plate_holder (Autodesk Fusion 360 design; units mm, degrees)
Autodesk Fusion 360 part; units mm, degrees
sketch "Sketch1" plane through (0, 0, 0) normal (0, 1, 0) x (1, 0, 0)
  line L0 (-177.8, -120.65) -> (0, -120.65)
  line L1 (0, -120.65) -> (0, 0)
  line L2 (0, 0) -> (-177.8, 0)
  line L3 (-177.8, 0) -> (-177.8, -120.65)
  circle A0 centre (-177.8, -120.65) radius 3.175
  circle A1 centre (-177.8, 0) radius 3.175
  circle A2 centre (0, 0) radius 3.175
  circle A3 centre (0, -120.65) radius 3.175
  line L4 (-158.9, -97.1) -> (-18.9, -97.1)
  line L5 (-18.9, -97.1) -> (-18.9, -72.1)
  line L6 (-18.9, -72.1) -> (-158.9, -72.1)
  line L7 (-158.9, -72.1) -> (-158.9, -97.1)
  line L8 (-158.9, -48.55) -> (-18.9, -48.55)
  line L9 (-18.9, -48.55) -> (-18.9, -23.55)
  line L10 (-18.9, -23.55) -> (-158.9, -23.55)
  line L11 (-158.9, -23.55) -> (-158.9, -48.55)
  line L12 (-180.975, -120.65) -> (-174.625, -120.65)
  line L13 (-174.625, -120.65) -> (-174.625, 0)
  line L14 (-174.625, 0) -> (-180.975, 0)
  line L15 (-180.975, 0) -> (-180.975, -120.65)
  line L16 (3.175, -120.65) -> (-3.175, -120.65)
  line L17 (-3.175, -120.65) -> (-3.175, 0)
  line L18 (-3.175, 0) -> (3.175, 0)
  line L19 (3.175, 0) -> (3.175, -120.65)
  line L20 (0, 0) -> (0, 3.175)
  line L21 (0, 3.175) -> (-177.8, 3.175)
  line L22 (-177.8, 3.175) -> (-177.8, -3.175)
  line L23 (-177.8, -3.175) -> (0, -3.175)
  line L24 (0, -3.175) -> (0, 3.175)
  line L25 (0, -120.65) -> (0, -123.825)
  line L26 (0, -123.825) -> (-177.8, -123.825)
  line L27 (-177.8, -123.825) -> (-177.8, -117.475)
  line L28 (-177.8, -117.475) -> (0, -117.475)
  line L29 (0, -117.475) -> (0, -123.825)
  line L30 (-177.8, -117.475) -> (-174.625, -117.475)
  line L31 (-174.625, -117.475) -> (-174.625, -120.65)
  line L32 (-174.625, -120.65) -> (-177.8, -120.65)
  line L33 (-177.8, -120.65) -> (-177.8, -117.475)
  line L34 (-158.9, -89.1) -> (-18.9, -89.1)
  line L35 (-18.9, -89.1) -> (-18.9, -80.1)
  line L36 (-18.9, -80.1) -> (-158.9, -80.1)
  line L37 (-158.9, -80.1) -> (-158.9, -89.1)
  line L38 (-150.9, -97.1) -> (-26.9, -97.1)
  line L39 (-26.9, -97.1) -> (-26.9, -72.1)
  line L40 (-26.9, -72.1) -> (-150.9, -72.1)
  line L41 (-150.9, -72.1) -> (-150.9, -97.1)
  line L42 (-177.8, -117.475) -> (-158.9, -89.1)
  line L43 (-174.625, -120.65) -> (-150.9, -97.1)
  line L44 (-26.9, -97.1) -> (-3.175, -120.65)
  line L45 (-18.9, -89.1) -> (0, -117.475)
  line L46 (-158.9, -40.55) -> (-18.9, -40.55)
  line L47 (-18.9, -40.55) -> (-18.9, -31.55)
  line L48 (-18.9, -31.55) -> (-158.9, -31.55)
  line L49 (-158.9, -31.55) -> (-158.9, -40.55)
  line L50 (-150.9, -48.55) -> (-26.9, -48.55)
  line L51 (-26.9, -48.55) -> (-26.9, -23.55)
  line L52 (-26.9, -23.55) -> (-150.9, -23.55)
  line L53 (-150.9, -23.55) -> (-150.9, -48.55)
  line L54 (-18.9, -31.55) -> (0, -3.175)
  line L55 (-26.9, -23.55) -> (-3.175, 0)
  line L56 (-158.9, -31.55) -> (-177.8, -3.175)
  line L57 (-150.9, -23.55) -> (-174.625, 0)
  line L58 (0, -60.325) -> (-177.8, -60.325)
  line L59 (-158.9, -40.55) -> (-174.625, -51.5608)
  line L60 (-150.9, -48.55) -> (-167.7164, -60.325)
  line L61 (-150.9, -72.1) -> (-167.7164, -60.325)
  line L62 (-158.9, -80.1) -> (-174.625, -69.0892)
  line L63 (-18.9, -80.1) -> (-3.175, -69.0892)
  line L64 (-18.9, -40.55) -> (-3.175, -51.5608)
  line L65 (-26.9, -48.55) -> (-10.0836, -60.325)
  line L66 (-26.9, -72.1) -> (-10.0836, -60.325)
  line L67 (-150.9, -97.1) -> (-130.6753, -117.475)
  line L68 (-136.8099, -97.1) -> (-116.5852, -117.475)
  line L69 (-116.5852, -117.475) -> (-101.3782, -97.1)
  line L70 (-26.9, -97.1) -> (-47.1247, -117.475)
  line L71 (-40.9901, -97.1) -> (-61.2148, -117.475)
  line L72 (-61.2148, -117.475) -> (-76.4218, -97.1)
  line L73 (-104.107, -117.475) -> (-88.9, -97.1)
  line L74 (-88.9, -97.1) -> (-73.693, -117.475)
  line L75 (-140.9, -72.1) -> (-18.4918, -54.4375)
  line L76 (-159.3082, -66.2125) -> (-36.9, -48.55)
  line L77 (-18.4918, -66.2125) -> (-140.9, -48.55)
  line L78 (-159.3082, -54.4375) -> (-36.9, -72.1)
  line L79 (-150.9, -23.55) -> (-130.6753, -3.175)
  line L80 (-136.8099, -23.55) -> (-116.5852, -3.175)
  line L81 (-116.5852, -3.175) -> (-101.3782, -23.55)
  line L82 (-104.107, -3.175) -> (-88.9, -23.55)
  line L83 (-88.9, -23.55) -> (-73.693, -3.175)
  line L84 (-61.2148, -3.175) -> (-76.4218, -23.55)
  line L85 (-40.9901, -23.55) -> (-61.2148, -3.175)
  line L86 (-26.9, -23.55) -> (-47.1247, -3.175)
  dimension "d1" = 177.8
  dimension "d2" = 120.65
  dimension "d3" = 6.35
  dimension "d4" = 6.35
  dimension "d6" = 6.35
  dimension "d7" = 6.35
  dimension "d10" = 25
  dimension "d11" = 25
  dimension "d12" = 140
  dimension "d13" = 140
  dimension "d14" = 23.55
  dimension "d15" = 23.55
  dimension "d16" = 18.9
  dimension "d17" = 18.9
  dimension "d18" = 8
  dimension "d19" = 8
  dimension "d20" = 8
  dimension "d21" = 8
  dimension "d22" = 8
  dimension "d23" = 8
  dimension "d24" = 8
  dimension "d25" = 8
  dimension "d26" = 125
  dimension "d27" = 125
  dimension "d28" = 10
  dimension "d30" = 45.212
  dimension "d31" = 45.212
  dimension "d32" = 10
  dimension "d33" = 10
  dimension "d34" = 10
  dimension "d35" = 10
  dimension "d36" = 10
  dimension "d37" = 10
  dimension "d38" = 10
  constraint horizontal L0
  constraint vertical L1
  constraint horizontal L2
  constraint vertical L3
  constraint coincident L1.end L2.start
  constraint coincident L0.start L3.end
  constraint coincident L2.end L3.start
  constraint coincident L0.end L1.start
  constraint horizontal L4
  constraint vertical L5
  constraint horizontal L6
  constraint vertical L7
  constraint horizontal L8
  constraint vertical L9
  constraint horizontal L10
  constraint vertical L11
  constraint horizontal L12
  constraint vertical L13
  constraint horizontal L14
  constraint vertical L15
  constraint coincident L2 L13.end
  constraint coincident A1 L13.end
  constraint coincident A0 L12.start
  constraint horizontal L16
  constraint vertical L17
  constraint horizontal L18
  constraint vertical L19
  constraint coincident A2 L17.end
  constraint coincident L2 L17.end
  constraint coincident A3 L16.start
  constraint perpendicular L2 L20
  constraint horizontal L21
  constraint vertical L22
  constraint horizontal L23
  constraint vertical L24
  constraint coincident A1 L22.end
  constraint coincident L3 L22.end
  constraint coincident A2 L20.end
  constraint coincident L20 L21.start
  constraint coincident A3 L25.end
  constraint perpendicular L0 L25
  constraint horizontal L26
  constraint vertical L27
  constraint horizontal L28
  constraint vertical L29
  constraint coincident A0 L27.end
  constraint coincident L3 L27.end
  constraint horizontal L30
  constraint vertical L31
  constraint horizontal L32
  constraint vertical L33
  constraint horizontal L34
  constraint vertical L35
  constraint horizontal L36
  constraint vertical L37
  constraint coincident L5 L35.end
  constraint coincident L7 L34.start
  constraint horizontal L38
  constraint vertical L39
  constraint horizontal L40
  constraint vertical L41
  constraint coincident L6 L39.end
  constraint coincident L4 L38.start
  constraint horizontal L46
  constraint vertical L47
  constraint horizontal L48
  constraint vertical L49
  constraint coincident L9 L47.end
  constraint coincident L11 L46.start
  constraint horizontal L50
  constraint vertical L51
  constraint horizontal L52
  constraint vertical L53
  constraint coincident L10 L51.end
  constraint coincident L8 L50.start
  constraint midpoint L1 L58.start
  constraint midpoint L3 L58.end
  constraint coincident L0.start L12
  constraint coincident L0.end L16
  constraint coincident L13 L59.end
  constraint coincident L58 L60.end
  constraint coincident L13 L62.end
  constraint parallel L61 L62
  constraint coincident L17 L63.end
  constraint parallel L60 L63
  constraint coincident L17 L64.end
  constraint parallel L62 L64
  constraint coincident L58 L65.end
  constraint parallel L64 L65
  constraint coincident L28 L67.end
  constraint perpendicular L43 L67
  constraint coincident L38 L68.start
  constraint coincident L28 L68.end
  constraint parallel L67 L68
  constraint coincident L4 L69.end
  constraint coincident L28 L70.end
  constraint coincident L38 L71.start
  constraint coincident L28 L71.end
  constraint coincident L4 L72.end
  constraint coincident L28 L73.start
  constraint midpoint L38 L73.end
  constraint coincident L28 L74.end
  constraint parallel L72 L74
  constraint parallel L70 L71
  constraint parallel L69 L73
  constraint coincident L40 L75.start
  constraint midpoint L65 L75.end
  constraint midpoint L61 L76.start
  constraint coincident L8 L76.end
  constraint midpoint L66 L77.start
  constraint coincident L50 L77.end
  constraint midpoint L60 L78.start
  constraint coincident L6 L78.end
  constraint symmetric L38.start L58 L52.end
  constraint symmetric L38.end L58 L51.end
  constraint symmetric L58 L67.end L79.end
  constraint symmetric L58 L68.start L80.start
  constraint symmetric L58 L68.end L80.end
  constraint symmetric L58 L69.end L81.end
  constraint symmetric L58 L70.end L86.end
  constraint symmetric L58 L71.start L85.start
  constraint symmetric L58 L71.end L84.start
  constraint symmetric L58 L72.end L84.end
  constraint symmetric L58 L73.start L82.start
  constraint symmetric L58 L73.end L82.end
  constraint symmetric L58 L74.end L83.end
  measures "d1" distance of L0.start L0.end
  measures "d2" distance of L0.start L2.end
  measures "d3" diameter of A0
  measures "d4" diameter of A3
  measures "d6" diameter of A2
  measures "d7" diameter of A1
  measures "d10" distance of L4.start L6.end
  measures "d11" distance of L8.start L10.end
  measures "d12" distance of L4.start L4.end
  measures "d13" distance of L8.start L8.end
  measures "d14" distance of L0 L4
  measures "d15" distance of L6 L8
  measures "d16" distance of L3 L7
  measures "d17" distance of L3 L11
  measures "d18" distance of L37 L41
  measures "d19" distance of L35 L39
  measures "d20" distance of L9 L51
  measures "d21" distance of L11 L53
  measures "d22" distance of L34 L38
  measures "d23" distance of L36 L40
  measures "d24" distance of L46 L50
  measures "d25" distance of L48 L52
  measures "d26" angle of L13 L62
  measures "d27" angle of L13 L59
  measures "d28" distance of L67 L68
  measures "d30" angle of L38 L70
  measures "d31" angle of L4 L67
  measures "d32" distance of L69 L73
  measures "d33" distance of L70 L71
  measures "d34" distance of L72 L74
  measures "d35" distance of L40.end L75.start
  measures "d36" distance of L50.end L76.end
  measures "d37" distance of L39.end L78.end
  measures "d38" distance of L50.start L77.end
extrude "Extrude1" add sketch "Sketch1" along normal blind 5 contours L0 L3 A0 L12 L27 L32 L33 | L3 A0 L12 L27 L33 | A0 L12 L27 | L0 A0 L12 L27 L32 | L0 L1 A3 L16 L29 | L0 A3 L16 L25 L29 | L3 A1 L14 L22 | A1 L14 L22 | A3 L16 L25 L29 | L1 A3 L16 L29 | L2 L3 A1 L14 L22 | L2 A1 L14 L22 | L2 A2 L18 L20 L24 | A2 L18 L20 L24 | L1 A2 L18 L24 | L1 L2 A2 L18 L24 makes body 1 at (3.1592, 1.6667, 0.3161) makes body 2 at (-176.3515, 3.3333, 2.8253) makes body 3 at (3.1592, 3.3333, 120.3339) makes body 4 at (-179.6534, 3.3333, 118.0721)
extrude "Extrude2" add sketch "Sketch1" 1 faces at (0.6951, 0, 119.3529) against normal blind 4 contours L0 L3 A0 L12 L27 L32 L33 | L3 A0 L12 L27 L33 | A0 L12 L27 | L0 A0 L12 L27 L32 | L0 L28 L43 L44 | L0 A0 A3 L26 | A0 L13 L28 L30 L31 | L13 L28 L31 L43 | L3 A0 A1 L15 | L13 L28 L30 L42 | L3 L13 L42 L58 | L0 L1 A3 L16 L29 | A3 L17 L28 | L0 A3 L16 L25 L29 | L17 L28 L44 | L4 L7 L13 L28 L42 L43 | L3 L13 L56 L58 | L3 A1 L14 L22 | A1 L14 L22 | A3 L16 L25 L29 | L1 A3 L16 L29 | L1 L17 L45 L58 | L1 A2 A3 L19 | L17 L28 L45 | L4 L5 L17 L28 L44 L45 | L4 L28 L38 L67 L68 | L4 L34 L38 L39 L41 | L4 L7 L34 L41 | L2 L3 A1 L14 L22 | A1 L13 L23 | L13 L23 L56 | L6 L7 L13 L58 L61 L62 | L8 L11 L13 L58 L59 L60 | L7 L34 L36 L37 L41 | L2 A1 A2 L21 | L2 A1 L14 L22 | L1 L17 L54 L58 | L4 L28 L38 L70 L71 | L4 L5 L34 L39 | L4 L28 L38 L69 L73 | L34 L36 L39 L41 | L13 L23 L57 | L2 L23 L55 L57 | L10 L11 L13 L23 L56 L57 | L6 L7 L36 L41 | L2 A2 L18 L20 L24 | A2 L18 L20 L24 | L1 A2 L18 L24 | L1 L2 A2 L18 L24 | A2 L17 L23 | L17 L23 L54 | L8 L9 L17 L58 L64 L65 | L5 L6 L17 L58 L63 L66 | L5 L34 L35 L36 L39 | L4 L28 L38 L72 L74 | L6 L36 L39 L40 L41 | L17 L23 L55 | L11 L46 L48 L49 L53 | L10 L11 L48 L53 | L8 L11 L46 L53 | L58 L76 L77 | L6 L40 L61 L75 L76 L78 | L8 L50 L60 L76 L77 L78 | L58 L75 L78 | L9 L10 L17 L23 L54 L55 | L5 L6 L36 L39 | L10 L23 L52 L79 L80 | L10 L48 L51 L52 L53 | L46 L48 L51 L53 | L8 L46 L50 L51 L53 | L6 L40 L66 L75 L77 L78 | L8 L50 L65 L75 L76 L77 | L9 L10 L48 L51 | L9 L46 L47 L48 L51 | L8 L9 L46 L51 | L10 L23 L52 L85 L86 | L10 L23 L52 L81 L82 | L10 L23 L52 L83 L84 on bodies 3 bodies 3 1 2 4
equation "d4 = d3"
equation "d6 = d3"
equation "d7 = d3"
equation "d11 = d10"
equation "d13 = d12"
equation "d15 = d14"
equation "d17 = d16"
equation "d19 = d18"
equation "d20 = d18"
equation "d21 = d18"
equation "d23 = d22"
equation "d24 = d22"
equation "d25 = d22"
equation "d27 = d26"
